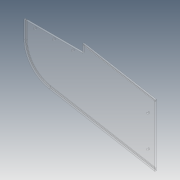
# Autodesk Inventor part: GE-12087-01
Saved by Autodesk Inventor 2012 (Build 160160000, 160)
## iProperties
Created: 2011-10-10
Part Number: GE-12087-01
Document SubType Name: Modeling
Designer: dfoster
Density: 1 g/cm^3
Description: Side
Material: Default
Title: Side
Author: dfoster
Autodesk Inventor part; units mm, degrees
ref_plane "YZ Plane" through (0, 0, 0) normal (1, 0, 0) x (0, 1, 0)
ref_plane "XZ Plane" through (0, 0, 0) normal (0, 1, 0) x (-1, 0, 0)
ref_plane "XY Plane" through (0, 0, 0) normal (0, 0, 1) x (1, 0, 0)
sketch "Sketch1" plane through (0, 0, 0) normal (0, 0, 1) x (1, 0, 0)
  line L0 (0, 0) -> (236.5375, 0)
  line L1 (527.05, 0) -> (527.05, 248.2464)
  line L2 (236.5375, 266.7) -> (0, 266.7)
  line L3 (0, 266.7) -> (0, 195.5132)
  line L4 (527.05, 0) -> (101.0217, 75.1203)
  line L5 (527.05, 248.2464) -> (236.5375, 299.4716)
  line L6 (236.5375, 266.7) -> (236.5375, 299.4716)
  arc A0 (0, 195.5132) -> (101.0217, 75.1203) centre (122.2502, 195.5132) ccw
  circle A1 centre (496.8875, 187.9214) radius 3.3655
  circle A2 centre (496.8875, 60.9214) radius 3.3655
  point P0 (0, 92.9331)
  dimension "d0" = 266.7
  dimension "d2" = 10
  dimension "d3" = 244.475
  dimension "d4" = 236.5375
  dimension "d5" = 527.05
  dimension "d18" = 122.2502
  dimension "d20" = 6.731
  dimension "d21" = 60.325
  dimension "d22" = 127
  dimension "d23" = 30.1625
  dimension "d24" = 30.1625
  constraints: 14 end point, 5 point on line, 4 parallel, 3 centre point, 2 point on circle, 2 tangent, 1 equal radius, 1 horizontal, 1 perpendicular
  measures "d0" distance of L2.end L0.start
  measures "d2" angle of L0 L4
  measures "d3" distance between parallel lines of L5 L4
  measures "d4" distance between parallel lines of L6 L3
  measures "d5" distance between parallel lines of L1 L3
  measures "d18" radius of A0
  measures "d20" diameter of A1
  measures "d21" vertical distance of L1.end A1.centre
  measures "d22" distance of A2.centre A1.centre
  measures "d23" distance from line of L1 A1.centre
  measures "d24" distance from line of L1 A2.centre
extrude "Extrusion1" add sketch "Sketch1" along normal blind 6.35 contours L4 A0 L3 L2 L6 L5 L1 | A1 | A2
sketch "Sketch2" plane through (0, 0, 0) normal (0, 0, -1) x (-1, 0, 0)
  line L0 (-527.05, 248.2464) -> (-236.5375, 299.4716) projected
  line L1 (-101.0217, 75.1203) -> (-527.05, 0) projected
  arc A0 (-101.0217, 75.1203) -> (0, 195.5132) centre (-122.2502, 195.5132) ccw projected
  line L2 (0, 266.7) -> (0, 195.5132) projected
  line L3 (-527.05, 243.4105) -> (-236.5375, 294.6356)
  line L4 (-527.05, 240.1865) -> (-236.5375, 291.4117)
  line L5 (-527.05, 4.836) -> (-101.8487, 79.8104)
  arc A1 (-101.8487, 79.8104) -> (-4.7625, 195.5132) centre (-122.2502, 195.5132) ccw
  line L6 (-4.7625, 195.5132) -> (-4.7625, 266.7)
  line L7 (-527.05, 8.0599) -> (-102.4, 82.9372)
  arc A2 (-102.4, 82.9372) -> (-7.9375, 195.5132) centre (-122.2502, 195.5132) ccw
  line L8 (-7.9375, 195.5132) -> (-7.9375, 266.7)
  line L9 (-527.05, 0) -> (-527.05, 248.2464) projected
  line L10 (-236.5375, 299.4716) -> (-236.5375, 266.7) projected
  line L11 (-236.5375, 266.7) -> (0, 266.7) projected
  line L12 (-527.05, 240.1865) -> (-527.05, 243.4105)
  line L13 (-236.5375, 294.6356) -> (-236.5375, 291.4117)
  line L14 (-7.9375, 266.7) -> (-4.7625, 266.7)
  line L15 (-527.05, 8.0599) -> (-527.05, 4.836)
  dimension "d27" = 4.7625
  dimension "d28" = 3.175
  dimension "d29" = 4.7625
  dimension "d30" = 4.7625
  dimension "d31" = 3.175
  dimension "d32" = 3.175
  constraints: 20 end point, 6 point on line, 4 point on circle, 3 collinear, 2 centre point, 2 parallel, 2 perpendicular, 2 other
  measures "d27" distance between parallel lines of L3 L0
  measures "d28" distance between parallel lines of L4 L3
  measures "d29" distance between parallel lines of L5 L1
  measures "d30" radial gap between concentric circles of A1 A0
  measures "d31" distance between parallel lines of L7 L5
  measures "d32" radial gap between concentric circles of A2 A1
extrude "Extrusion2" cut sketch "Sketch2" against normal blind 3.175 contours L3 L10 L4 L9 | L7 A2 L8 L11 L6 A1 L5 L9
extrude "Extrusion3" cut sketch "Sketch1" along normal blind 25.4 contours A1 | A2
hole "Hole1" at (41.275, 254, 0) direction (0, 0, 1) diameter 6.731 depth 25.4 tip angle 118
pattern_linear "Rectangular Pattern1" count 3 spacing 76.2 along (1, 0, 0) of "Hole1"
equation "\"d24\" = d23"
equation "\"d29\" = d27"
equation "\"d30\" = d27"
body "Solid1"
